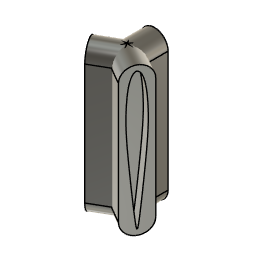
finHolder v2 (Autodesk Fusion 360 design; units mm, degrees)
Autodesk Fusion 360 part; units mm, degrees
sketch "Sketch1" plane through (0, 0, 0) normal (0, 1, 0) x (1, 0, 0)
  line L0 (-5, 0) -> (5, 0)
  line L1 (5, 0) -> (5, -54)
  line L2 (5, -54) -> (-5, -54)
  line L3 (-5, -54) -> (-5, 0)
  dimension "d1" = 10
  dimension "d2" = 54
  dimension "d3" = 5
  constraint horizontal L0
  constraint vertical L1
  constraint horizontal L2
  constraint vertical L3
  constraint horizontal origin L0.end
  measures "d1" distance of L0.start L0.end
  measures "d2" distance of L0.start L2.end
  measures "d3" distance of origin L0.end
extrude "Extrude1" add sketch "Sketch1" along normal blind 10 makes body 1
sketch "Sketch2" plane through (0, 10, 0) normal (0, 1, 0) x (-1, 0, 0)
  line L0 (5, 54) -> (-5, 54)
  line L1 (-5, 54) -> (-5, 0)
  line L2 (-5, 0) -> (5, 0)
  line L3 (5, 0) -> (5, 54)
  spline S0 degree 5 poles (0, 2) (0.0829, 2) (0.2486, 2.4125) (0.5186, 4.2686) (1.0074, 8.9269) (1.7486, 16.855) (2.4545, 25.0304) (2.9459, 32.0654) (3.0612, 37.1221) (2.9371, 41.6893) (2.5475, 46.8402) (1.6202, 51.0987) (0, 52.8664) (-1.6202, 51.0987) (-2.5475, 46.8402) (-2.9371, 41.6893) (-3.0612, 37.1221) (-2.9459, 32.0654) (-2.4545, 25.0304) (-1.7486, 16.855) (-1.0074, 8.9269) (-0.5186, 4.2686) (-0.2486, 2.4125) (-0.0829, 2) (0, 2) knots 0 0 0 0 0 0 0.05 0.1 0.15 0.2 0.25 0.3 0.35 0.4 0.45 0.5 0.55 0.6 0.65 0.7 0.75 0.8 0.85 0.9 0.95 1 1 1 1 1 1
  line L4 (3, 32) -> (3, 42)
  line L5 (-3, 42) -> (-3, 32)
  line L6 (1.5, 52) -> (-1.5, 52)
  line L7 (-0.25, 2) -> (0.25, 2)
  point P0 (3, 37)
  point P1 (0, 52)
  point P2 (-3, 37)
  dimension "d13" = 35
  dimension "d14" = 15
  dimension "d15" = 0.5
  dimension "d16" = 3
  dimension "d17" = 10
  dimension "d18" = 6
  dimension "d19" = 3
  dimension "d20" = 2
  constraint horizontal P0 P2
  constraint midpoint P0 L4
  constraint vertical L4
  constraint midpoint P2 L5
  constraint vertical L5
  constraint midpoint P1 L6
  constraint horizontal L6
  constraint midpoint S0.start L7
  constraint horizontal L7
  constraint equal L4 L5
  constraint vertical origin S0.start
  constraint vertical origin P1
  measures "d13" distance of S0.start P2
  measures "d14" vertical distance of P1 P2
  measures "d15" distance of L7.start L7.end
  measures "d16" distance of L6.start L6.end
  measures "d17" distance of L4.start L4.end
  measures "d18" distance of P0 P2
  measures "d19" horizontal distance of P0 P1
  measures "d20" distance of origin S0.start
extrude "Extrude2" cut sketch "Sketch2" against normal blind 5 contours S0 bodies 1
pattern_circular "C-Pattern1" count 3 over 360 about axis through (0, 0, 1.75) along (0, 0, 1) of bodies 1 makes body 2 at (0.8333, -1.4434, 18) makes body 3 at (0.8333, 1.4434, 18)
fillet "Fillet1" radius 5 12 edges at (5, 5, 54) (-5, 5, 54) (5, 5, 0) (-5, 5, 0) (-6.8301, 1.8301, 54) (-1.8301, -6.8301, 54) (-1.8301, -6.8301, 0) (-6.8301, 1.8301, 0) (6.8301, 1.8301, 54) (1.8301, -6.8301, 54) (1.8301, -6.8301, 0) (6.8301, 1.8301, 0) on bodies 1 2 3
